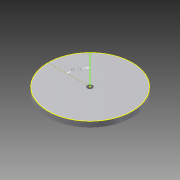
# Autodesk Inventor part: 后轮
Saved by Autodesk Inventor 2013 (Build 170138000, 138)
## iProperties
Created: 2012-10-03
Part Number: 后轮
Material: PVC 管
Document SubType Name: Modeling
Designer: Zhensheng
Density: 1 g/cm^3
Author: Zhensheng
Autodesk Inventor part; units mm, degrees
ref_plane "YZ Plane" through (0, 0, 0) normal (1, 0, 0) x (0, 1, 0)
ref_plane "XZ Plane" through (0, 0, 0) normal (0, 1, 0) x (-1, 0, 0)
ref_plane "XY Plane" through (0, 0, 0) normal (0, 0, 1) x (1, 0, 0)
sketch "草图1" plane through (0, 0, 0) normal (0, 0, 1) x (1, 0, 0)
  circle A0 centre (0, 0) radius 75
  circle A1 centre (0, 0) radius 5
  dimension "后轮直径" = 150
  dimension "孔直径" = 10
  constraints: 2 centre point, 2 coincident
  measures "后轮直径" diameter of A0
  measures "孔直径" diameter of A1
extrude "拉伸1" add sketch "草图1" along normal mid plane 10
sketch "草图2" plane through (0, 0, 5) normal (0, 0, 1) x (1, 0, 0)
  circle A0 centre (0, 0) radius 75 projected
  line L0 (0, 0) -> (-53.033, 53.033)
  line L1 (0, 0) -> (-75, 0) construction
  constraints: 4 end point, 2 point on circle
